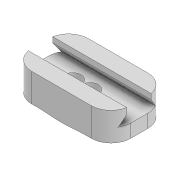
# Autodesk Inventor part: Porta herramientas p2
Saved by Autodesk Inventor 2022 (Build 260153000, 153)
## iProperties
Created: 2022-10-25
Part Number: Porta herramientas p2
Material: Generic
Document SubType Name: Modeling
Designer: ADMIN
Density: 1 g/cm^3
Appearance: Default
Author: ADMIN
## iProperties of the stored document Porta herramientas p2_3DPrint.ipt
Created: 2022-10-25
Part Number: Porta herramientas p2_3DPrint
Material: Generic
Document SubType Name: Modeling
Designer: ADMIN
Density: 1 g/cm^3
Appearance: Default
Author: ADMIN
Autodesk Inventor part; units mm, degrees
ref_plane "YZ Plane" through (0, 0, 0) normal (1, 0, 0) x (0, 1, 0)
ref_plane "XZ Plane" through (0, 0, 0) normal (0, 1, 0) x (-1, 0, 0)
ref_plane "XY Plane" through (0, 0, 0) normal (0, 0, 1) x (1, 0, 0)
sketch "Sketch1" plane through (0, 0, 0) normal (0, 1, 0) x (-1, 0, 0)
  ellipse E0 centre (0, 0) end of major axis (-10.7821, 0) minor radius 7.6241 (0, 7.6241) -> (0, -7.6241) ccw
  spline S0 degree 3 poles (0, 7.6241) (0.5874, 7.6036) (1.2899, 7.5399) (2.4433, 7.368) (3.1227, 7.2268) (4.2258, 6.9261) (4.8681, 6.7085) (5.9026, 6.2778) (6.4991, 5.9807) (7.5188, 5.3684) (8.084, 4.9623) (9.0956, 4.0283) (9.5409, 3.4991) (10.1481, 2.5291) (10.4057, 1.9733) (10.6833, 1.0314) (10.7665, 0.4716) (10.7665, 0) (10.7665, -0.4716) (10.6833, -1.0314) (10.4057, -1.9733) (10.1481, -2.5291) (9.5409, -3.4991) (9.0956, -4.0283) (8.084, -4.9623) (7.5188, -5.3684) (6.4991, -5.9807) (5.9026, -6.2778) (4.8681, -6.7085) (4.2258, -6.9261) (3.1227, -7.2268) (2.4433, -7.368) (1.2899, -7.5399) (0.5874, -7.6036) (0, -7.6241) knots -1.249592 -1.249592 -1.249592 -1.249592 -1.087686 -1.087686 -0.928403 -0.928403 -0.772743 -0.772743 -0.619768 -0.619768 -0.44513 -0.44513 -0.270492 -0.270492 -0.129899 -0.129899 0 0 0 0.129899 0.129899 0.270492 0.270492 0.44513 0.44513 0.619768 0.619768 0.772743 0.772743 0.928403 0.928403 1.087686 1.087686 1.249592 1.249592 1.249592 1.249592
  circle A0 centre (6.5349, 0) radius 1.6337
  circle A1 centre (0, 0) radius 1.6337
  spline S1 degree 3 poles (0, 7.6241) (0.5874, 7.6036) (1.2899, 7.5399) (2.4433, 7.368) (3.1227, 7.2268) (4.2258, 6.9261) (4.8681, 6.7085) (5.9026, 6.2778) (6.4991, 5.9807) (7.5188, 5.3684) (8.084, 4.9623) (9.0956, 4.0283) (9.5409, 3.4991) (10.1481, 2.5291) (10.4057, 1.9733) (10.6833, 1.0314) (10.7665, 0.4716) (10.7665, 0) (10.7665, -0.4716) (10.6833, -1.0314) (10.4057, -1.9733) (10.1481, -2.5291) (9.5409, -3.4991) (9.0956, -4.0283) (8.084, -4.9623) (7.5188, -5.3684) (6.4991, -5.9807) (5.9026, -6.2778) (4.8681, -6.7085) (4.2258, -6.9261) (3.1227, -7.2268) (2.4433, -7.368) (1.2899, -7.5399) (0.5874, -7.6036) (0, -7.6241) knots -1.249592 -1.249592 -1.249592 -1.249592 -1.087686 -1.087686 -0.928403 -0.928403 -0.772743 -0.772743 -0.619768 -0.619768 -0.44513 -0.44513 -0.270492 -0.270492 -0.129899 -0.129899 0 0 0 0.129899 0.129899 0.270492 0.270492 0.44513 0.44513 0.619768 0.619768 0.772743 0.772743 0.928403 0.928403 1.087686 1.087686 1.249592 1.249592 1.249592 1.249592
  ellipse E1 centre (0, 0) end of major axis (-10.7821, 0) minor radius 7.6241 (0, 7.6241) -> (0, -7.6241) ccw
  ellipse E2 centre (0, 0) end of major axis (12, 0) minor radius 9
  point P0 (33.8865, 0)
  dimension "d0" = 12
  dimension "d1" = 9
  constraints: 3 centre point, 1 coincident, 13 other
extrude "Extrusion1" add sketch "Sketch1" along normal blind 1 contours E2
sketch "Sketch2" plane through (0, 1, 0) normal (0, 1, 0) x (1, 0, 0)
  line L0 (17.5, -10) -> (-17.5, -10)
  line L1 (-17.5, -10) -> (-17.5, 10)
  line L2 (-17.5, 10) -> (17.5, 10)
  line L3 (17.5, 10) -> (17.5, -10)
  line L4 (17.5, -10) -> (-17.5, 10) construction
  line L5 (-17.5, -10) -> (17.5, 10) construction
  point P0 (0, 0)
  dimension "d4" = 35
  dimension "d5" = 20
  constraints: 12 end point, 2 midpoint, 2 parallel, 1 horizontal, 1 perpendicular
  measures "d4" distance of L1.end L2.end
  measures "d5" distance of L0.end L1.end
extrude "Extrusion2" add sketch "Sketch2" along normal blind 5
sketch "Sketch3" plane through (0, 0, 0) normal (0, 1, 0) x (-1, 0, 0)
  ellipse E0 centre (0, 0) end of major axis (-9.8995, 0) minor radius 7 (0, 7) -> (0, -7) ccw
  spline S0 degree 3 poles (0, 7) (0.5394, 6.9812) (1.1843, 6.9227) (2.2433, 6.7649) (2.8671, 6.6353) (3.8799, 6.3592) (4.4696, 6.1593) (5.4194, 5.7639) (5.9671, 5.4911) (6.9033, 4.9289) (7.4222, 4.5561) (8.3511, 3.6986) (8.76, 3.2127) (9.3175, 2.322) (9.554, 1.8118) (9.8088, 0.9469) (9.8852, 0.433) (9.8852, 0) (9.8852, -0.433) (9.8088, -0.9469) (9.554, -1.8118) (9.3175, -2.322) (8.76, -3.2127) (8.3511, -3.6986) (7.4222, -4.5561) (6.9033, -4.9289) (5.9671, -5.4911) (5.4194, -5.7639) (4.4696, -6.1593) (3.8799, -6.3592) (2.8671, -6.6353) (2.2433, -6.7649) (1.1843, -6.9227) (0.5394, -6.9812) (0, -7) knots -1.249592 -1.249592 -1.249592 -1.249592 -1.087686 -1.087686 -0.928403 -0.928403 -0.772743 -0.772743 -0.619768 -0.619768 -0.44513 -0.44513 -0.270492 -0.270492 -0.129899 -0.129899 0 0 0 0.129899 0.129899 0.270492 0.270492 0.44513 0.44513 0.619768 0.619768 0.772743 0.772743 0.928403 0.928403 1.087686 1.087686 1.249592 1.249592 1.249592 1.249592
  circle A0 centre (6, 0) radius 1.5
  circle A1 centre (0, 0) radius 1.5
  spline S1 degree 3 poles (0, 7) (0.5394, 6.9812) (1.1843, 6.9227) (2.2433, 6.7649) (2.8671, 6.6353) (3.8799, 6.3592) (4.4696, 6.1593) (5.4194, 5.7639) (5.9671, 5.4911) (6.9033, 4.9289) (7.4222, 4.5561) (8.3511, 3.6986) (8.76, 3.2127) (9.3175, 2.322) (9.554, 1.8118) (9.8088, 0.9469) (9.8852, 0.433) (9.8852, 0) (9.8852, -0.433) (9.8088, -0.9469) (9.554, -1.8118) (9.3175, -2.322) (8.76, -3.2127) (8.3511, -3.6986) (7.4222, -4.5561) (6.9033, -4.9289) (5.9671, -5.4911) (5.4194, -5.7639) (4.4696, -6.1593) (3.8799, -6.3592) (2.8671, -6.6353) (2.2433, -6.7649) (1.1843, -6.9227) (0.5394, -6.9812) (0, -7) knots -1.249592 -1.249592 -1.249592 -1.249592 -1.087686 -1.087686 -0.928403 -0.928403 -0.772743 -0.772743 -0.619768 -0.619768 -0.44513 -0.44513 -0.270492 -0.270492 -0.129899 -0.129899 0 0 0 0.129899 0.129899 0.270492 0.270492 0.44513 0.44513 0.619768 0.619768 0.772743 0.772743 0.928403 0.928403 1.087686 1.087686 1.249592 1.249592 1.249592 1.249592
  ellipse E1 centre (0, 0) end of major axis (-9.8995, 0) minor radius 7 (0, 7) -> (0, -7) ccw
  point P0 (31.1127, 0)
  constraints: 2 centre point, 12 other
extrude "Extrusion3" cut sketch "Sketch3" along normal blind 3 contours A0 | A1
sketch "Sketch4" plane through (0, 6, 0) normal (0, 1, 0) x (1, 0, 0)
  circle A0 centre (-6, 0) radius 1.5 projected
  circle A1 centre (0, 0) radius 1.5 projected
  circle A2 centre (-6, 0) radius 3
  circle A3 centre (0, 0) radius 3
  point P0 (-3, 0)
  dimension "d10" = 6
  dimension "d11" = 6
  constraints: 2 centre point, 2 coincident
  measures "d10" diameter of A2
  measures "d11" diameter of A3
extrude "Extrusion4" cut sketch "Sketch4" against normal blind 3 contours A0 | A1 | A2 | A3
fillet "Fillet1" radius 7 4 edges at (17.5, 3.5, -10) (17.5, 3.5, 10) (-17.5, 3.5, -10) (-17.5, 3.5, 10)
fillet "Fillet2" radius 5 1 edges at (12, 1, 0)
sketch "Sketch5" plane through (0, 6, 0) normal (0, 1, 0) x (1, 0, 0)
  arc A0 (-17.5, -3) -> (-10.5, -10) centre (-10.5, -3) ccw projected
  line L0 (-10.5, -10) -> (10.5, -10) projected
  arc A1 (10.5, -10) -> (17.5, -3) centre (10.5, -3) ccw projected
  line L1 (17.5, -3) -> (17.5, 3) projected
  arc A2 (17.5, 3) -> (10.5, 10) centre (10.5, 3) ccw projected
  line L2 (10.5, 10) -> (-10.5, 10) projected
  arc A3 (-10.5, 10) -> (-17.5, 3) centre (-10.5, 3) ccw projected
  line L3 (-17.5, 3) -> (-17.5, -3) projected
  circle A4 centre (-6, 0) radius 3 projected
  circle A5 centre (0, 0) radius 3 projected
  line L4 (21.6457, 4) -> (-21.7327, 4)
  line L5 (21.6457, -4) -> (-21.7327, -4)
  point P0 (-3, 0)
  point P1 (17.4282, -4)
  point P2 (-17.4282, -4)
  point P3 (-17.4282, 4)
  point P4 (17.4282, 4)
  dimension "d16" = 6
  dimension "d17" = 6
  constraints: 4 end point, 2 horizontal, 2 horizontal alignment
  measures "d16" distance between parallel lines of L4 L2
  measures "d17" distance between parallel lines of L0 L5
extrude "Extrusion5" add sketch "Sketch5" along normal blind 5 contours L5 A1 L0 A0 | A3 L2 A2 L4
sketch "Sketch6" plane through (-17.5, 1, -3) normal (-1, 0, 0) x (0, 0, 1)
  line L0 (13, 10) -> (7, 10) projected
  line L1 (0, 5) -> (6, 5) projected
  line L2 (7, 5) -> (7, 10) projected
  line L3 (-3, 5) -> (9, 5)
  line L4 (-3, 5) -> (-1, 8)
  line L5 (7, 8) -> (9, 5)
  line L6 (-1, 5) -> (-1, 10) projected
  line L7 (-1, 8) -> (7, 8)
  point P0 (3, -1)
  point P1 (3, 5)
  dimension "d21" = 3
  dimension "d22" = 3
  dimension "d23" = 0
  dimension "d24" = 2
  dimension "d25" = 2
  dimension "d31" = 8
  constraints: 8 end point, 1 horizontal, 1 perpendicular, 1 point on line
  measures "d21" distance of L6.start L4.end
  measures "d22" distance from line of L3 L5.start
  measures "d23" distance between parallel lines of L1 L3
  measures "d24" distance from line of L6 L3.start
  measures "d25" distance from line of L2 L3.end
  measures "d31" distance between parallel lines of L2 L6
extrude "Extrusion6" cut sketch "Sketch6" against normal blind 36.5
sketch "Sketch7" plane through (0, 0, 0) normal (0, -1, 0) x (1, 0, 0)
  ellipse E0 centre (0, 0) end of major axis (-12, 0) minor radius 9 projected
  ellipse E1 centre (0, 0) end of major axis (-10.7821, 0) minor radius 7.6241 (0, -7.6241) -> (0, 7.6241) ccw projected
  circle A0 centre (0, 0) radius 1.5 projected
  ellipse E2 centre (0, 0) end of major axis (-11.4484, 0) minor radius 8.1464
  line L0 (-10.7665, 0) -> (-9.4974, 0.7747)
  point P0 (12, 0.0028)
  constraints: 2 end point, 1 coincident, 6 other
sketch "Sketch8" plane through (17.5, 1, 3) normal (1, 0, 0) x (0, 0, -1)
  line L0 (0, 5) -> (6, 5) projected
  line L1 (9, 5) -> (7, 8) projected
  line L2 (6, 5) -> (9, 5) projected
  line L3 (-3, 5) -> (0, 5) projected
  line L4 (-1, 8) -> (-3, 5) projected
  line L5 (-1, 8) -> (-1, 10) projected
  line L6 (7, 8) -> (7, 10) projected
  line L7 (7, 10) -> (7, 8)
  line L8 (7, 8) -> (9, 5)
  line L9 (-3, 5) -> (-1, 8)
  line L10 (-1, 10.1812) -> (-1, 8)
  line L11 (-1, 10) -> (-7, 10) projected
  line L12 (-3, 5) -> (9, 5)
  line L13 (7, 10) -> (-1, 10)
  line L14 (7.3, 10) -> (7.3, 8.0908)
  line L15 (7.3, 8.0908) -> (9.5606, 4.7)
  line L16 (9.5606, 4.7) -> (6, 4.7)
  line L17 (6, 4.7) -> (0, 4.7)
  line L18 (0, 4.7) -> (-3.5606, 4.7)
  line L19 (-3.5606, 4.7) -> (-1.3, 8.0908)
  line L20 (-1.3, 8.0908) -> (-1.3, 9.7)
  line L21 (-1.3, 9.7) -> (-7, 9.7)
  line L22 (7.3, 10) -> (6.9353, 10)
  line L23 (-1.3, 9.7) -> (-1.3, 10)
  line L24 (-1, 10) -> (-1.3, 10)
  point P0 (3, -1)
  dimension "d28" = 0.3
  constraints: 34 end point, 4 perpendicular, 3 point on line, 2 collinear, 2 vertical, 7 other
  measures "d28" distance between parallel lines of L2 L16
extrude "Extrusion7" cut sketch "Sketch8" against normal blind 38 contours L0 L2 L1 L6 L22 L14 L15 L16 L17 L18 L19 L20 L23 L11 L5 L4 L3
equation "\"d22\" = d21"
equation "\"d25\" = d24"
body "Solid1"
